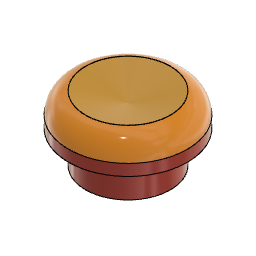
fidget_holder (Autodesk Fusion 360 design; units mm, degrees)
Autodesk Fusion 360 part; units mm, degrees
sketch "Sketch1" plane through (0, 0, 0) normal (0, 0, 1) x (1, 0, 0)
  circle A0 centre (0, 0) radius 3.925
  dimension "d1" = 7.85
  constraint coincident A0.centre origin
  measures "d1" diameter of A0
extrude "Extrude1" add sketch "Sketch1" against normal blind 3 makes body 1
sketch "Sketch2" plane through (0, 0, 0) normal (0, 0, 1) x (-1, 0, 0)
  circle A0 centre (0, 0) radius 3.925
  circle A1 centre (0, 0) radius 5.5
  dimension "d4" = 11
  constraint coincident A0.centre A1.centre
  measures "d4" diameter of A1
extrude "Extrude2" add sketch "Sketch2" along normal blind 3 separate body makes body 2
sketch "Sketch3" plane through (0, 0, 0) normal (1, 0, 0) x (0, 1, 0)
  line L0 (4, 3) -> (0, 2)
  line L1 (0, 2) -> (0, 0)
  line L2 (0, 0) -> (4, 0)
  line L3 (4, 0) -> (4, 3)
  dimension "d7" = 4
  dimension "d8" = 3
  dimension "d9" = 2
  constraint coincident L1.end L2.start
  constraint vertical L1
  constraint perpendicular L1 L2
  constraint perpendicular L2 L3
  measures "d7" horizontal distance of L0.start L0.end
  measures "d8" distance of L0.start L2.end
  measures "d9" distance of L0.end L1.end
revolve "Revolve1" add sketch "Sketch3" angle 360 about axis through (0, 0, 0) along (0, 0, -1) bodies 2 1
fillet "Fillet1" radius 2 1 edges at (5.1278, 1.9889, 3) on bodies 2
